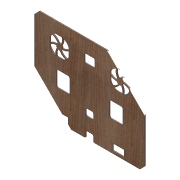
# Autodesk Inventor part: BackCover
Saved by Autodesk Inventor 2015 (Build 190159000, 159)
## iProperties
Created: 2018-04-12
Part Number: BackCover
Material: Wood (Birch)
Document SubType Name: Modeling
Designer: Ghassan Yusuf
Density: 0.55 g/cm^3
Appearance: Birch - Natural Polished
Author: Ghassan Yusuf
Autodesk Inventor part; units mm, degrees
ref_plane "YZ Plane" through (0, 0, 0) normal (1, 0, 0) x (0, 1, 0)
ref_plane "XZ Plane" through (0, 0, 0) normal (0, 1, 0) x (-1, 0, 0)
ref_plane "XY Plane" through (0, 0, 0) normal (0, 0, 1) x (1, 0, 0)
sketch "80 mm Cooling Fan Cut Template" plane through (0, 0, 0) normal (0, 0, 1) x (1, 0, 0)
  line L0 (-145.6797, 134) -> (-114.1203, 134)
  line L1 (-89.9, 109.7797) -> (-89.9, 78.2203)
  line L2 (-114.1203, 54) -> (-145.6797, 54)
  line L3 (-169.9, 78.2203) -> (-169.9, 109.7797)
  circle A0 centre (-165.65, 129.75) radius 2.35
  circle A1 centre (-94.15, 129.75) radius 2.35
  circle A2 centre (-165.65, 58.25) radius 2.35
  circle A3 centre (-94.15, 58.25) radius 2.35
  arc A4 (-89.9, 109.7797) -> (-114.1203, 134) centre (-129.9, 94) ccw
  arc A5 (-145.6797, 134) -> (-169.9, 109.7797) centre (-129.9, 94) ccw
  arc A6 (-169.9, 78.2203) -> (-145.6797, 54) centre (-129.9, 94) ccw
  arc A7 (-114.1203, 54) -> (-89.9, 78.2203) centre (-129.9, 94) ccw
  point P0 (-127.7378, 96.1622)
  point P1 (-129.9, 134)
  point P2 (-89.9, 94)
  dimension "d46" = 4.7
  dimension "d47" = 71.5
  dimension "d48" = 71.5
  dimension "d49" = 4.25
  dimension "d50" = 4.25
  dimension "d52" = 80
  dimension "d53" = 80
  measures "d46" diameter of A0
  measures "d47" distance of A1.centre A0.centre
  measures "d48" distance of A2.centre A0.centre
  measures "d49" distance from line of L0 A0.centre
  measures "d50" distance from line of L3 A0.centre
  measures "d52" distance between parallel lines of L1 L3
  measures "d53" distance between parallel lines of L2 L0
sketch "Faces Holing" plane through (0, 0, 0) normal (0, 0, 1) x (1, 0, 0)
  circle A0 centre (-222, 150) radius 3
  circle A1 centre (-222, 5) radius 3
  circle A2 centre (-222, -150) radius 3
  circle A3 centre (222, -150) radius 3
  circle A4 centre (222, 5) radius 3
  circle A5 centre (222, 150) radius 3
  circle A6 centre (0, 160) radius 3
  circle A7 centre (0, -150) radius 3
  point P0 (0, 2.5)
  dimension "d60" = 6
  dimension "d61" = 145
  dimension "d62" = 155
  measures "d60" diameter of A0
  measures "d61" distance of A4.centre A5.centre
  measures "d62" distance of A3.centre A4.centre
sketch "80 mm Cooling Fan Cut Template_1" plane through (0, 0, 0) normal (0, 0, 1) x (1, 0, 0)
  arc A0 (-145.6797, 134) -> (-169.9, 109.7797) centre (-129.9, 94) ccw
  arc A1 (-114.1203, 54) -> (-89.9, 78.2203) centre (-129.9, 94) ccw
  circle A2 centre (-165.65, 129.75) radius 2.35
  circle A3 centre (-94.15, 129.75) radius 2.35
  circle A4 centre (-165.65, 58.25) radius 2.35
  circle A5 centre (-94.15, 58.25) radius 2.35
  arc A6 (-98.8905, 123.7895) -> (-123.8985, 104.965) centre (-90.5696, 86.7117) ccw
  arc A7 (-102.3594, 127.023) -> (-127.7177, 106.308) centre (-90.5696, 86.7117) ccw
  arc A8 (-140.1937, 135.7497) -> (-136.3952, 104.68) centre (-103.9229, 124.417) ccw
  arc A9 (-144.7285, 134.3623) -> (-139.4679, 102.0439) centre (-103.9229, 124.417) ccw
  arc A10 (-171.2032, 105.9602) -> (-142.3967, 93.7149) centre (-143.2534, 131.7053) ccw
  arc A11 (-172.269, 101.3393) -> (-141.6502, 89.7359) centre (-143.2534, 131.7053) ccw
  arc A12 (-160.9095, 64.2105) -> (-135.9015, 83.035) centre (-169.2304, 101.2883) ccw
  arc A13 (-157.4406, 60.977) -> (-132.0823, 81.692) centre (-169.2304, 101.2883) ccw
  arc A14 (-119.6063, 52.2503) -> (-123.4048, 83.32) centre (-155.8771, 63.583) ccw
  arc A15 (-115.0715, 53.6377) -> (-120.3321, 85.9561) centre (-155.8771, 63.583) ccw
  arc A16 (-88.5968, 82.0398) -> (-117.4033, 94.2851) centre (-116.5466, 56.2947) ccw
  arc A17 (-87.531, 86.6607) -> (-118.1498, 98.2641) centre (-116.5466, 56.2947) ccw
  arc A18 (-89.9, 109.7797) -> (-98.8905, 123.7895) centre (-129.9, 94) ccw
  arc A19 (-102.3594, 127.023) -> (-114.1203, 134) centre (-129.9, 94) ccw
  line L0 (-145.6797, 134) -> (-144.8151, 134)
  line L1 (-140.6948, 134) -> (-114.1203, 134)
  line L2 (-169.9, 78.2203) -> (-169.9, 99.2406)
  line L3 (-169.9, 104.6137) -> (-169.9, 109.7797)
  arc A20 (-169.9, 78.2203) -> (-160.9095, 64.2105) centre (-129.9, 94) ccw
  arc A21 (-157.4406, 60.977) -> (-145.6797, 54) centre (-129.9, 94) ccw
  line L4 (-114.1203, 54) -> (-114.9849, 54)
  line L5 (-119.1052, 54) -> (-145.6797, 54)
  line L6 (-89.9, 109.7797) -> (-89.9, 88.7594)
  line L7 (-89.9, 83.3863) -> (-89.9, 78.2203)
  arc A22 (-118.1498, 98.2641) -> (-123.8985, 104.965) centre (-129.9, 94) ccw
  arc A23 (-127.7177, 106.308) -> (-136.3952, 104.68) centre (-129.9, 94) ccw
  arc A24 (-139.4679, 102.0439) -> (-142.3967, 93.7149) centre (-129.9, 94) ccw
  arc A25 (-141.6502, 89.7359) -> (-135.9015, 83.035) centre (-129.9, 94) ccw
  arc A26 (-132.0823, 81.692) -> (-123.4048, 83.32) centre (-129.9, 94) ccw
  arc A27 (-120.3321, 85.9561) -> (-117.4033, 94.2851) centre (-129.9, 94) ccw
  point P0 (-127.7378, 96.1622)
  point P1 (-129.9, 134)
  point P2 (-89.9, 94)
  dimension "d88" = 4.7
  dimension "d89" = 71.5
  dimension "d90" = 71.5
  dimension "d104" = 4
  dimension "d107" = 360
  measures "d88" diameter of A2
  measures "d89" distance of A3.centre A2.centre
  measures "d90" distance of A4.centre A2.centre
  measures "d104" radial gap between concentric circles of A6 A7
sketch "Sketch1" plane through (0, 0, 0) normal (0, 0, 1) x (1, 0, 0)
  line L0 (-230, 180) -> (230, 180)
  line L1 (230, 180) -> (230, -180)
  line L2 (230, -180) -> (-230, -180)
  line L3 (-230, -180) -> (-230, 180)
  line L4 (-21.9, 125) -> (21.9, 125)
  line L5 (21.9, 125) -> (21.9, 89)
  line L6 (21.9, 89) -> (-21.9, 89)
  line L7 (-21.9, 89) -> (-21.9, 125)
  line L8 (-139.5, 8) -> (-82.5, 8)
  line L9 (-82.5, 8) -> (-82.5, -58.6)
  line L10 (-82.5, -58.6) -> (-139.5, -58.6)
  line L11 (-139.5, -58.6) -> (-139.5, 8)
  line L12 (82.5, 8) -> (139.5, 8)
  line L13 (139.5, 8) -> (139.5, -58.6)
  line L14 (139.5, -58.6) -> (82.5, -58.6)
  line L15 (82.5, -58.6) -> (82.5, 8)
  line L16 (-16.075, -71) -> (16.075, -71)
  line L17 (16.075, -71) -> (16.075, -100.45)
  line L18 (16.075, -100.45) -> (-16.075, -100.45)
  line L19 (-16.075, -100.45) -> (-16.075, -71)
  point P0 (0, 0)
  point P1 (0, 180)
  point P2 (-230, 0)
  point P3 (0, 125)
  point P4 (0, -71)
  point P5 (0, -147)
  dimension "d0" = 460
  dimension "d1" = 360
  dimension "d2" = 55
  dimension "d3" = 43.8
  dimension "d4" = 36
  dimension "d5" = 29.45
  dimension "d6" = 32.15
  dimension "d7" = 66.6
  dimension "d8" = 57
  dimension "d9" = 172
  dimension "d10" = 165
  dimension "d11" = 160
  dimension "d41" = 82.5
  constraints: 40 end point, 10 parallel, 5 horizontal, 5 perpendicular, 4 midpoint, 4 vertical alignment, 2 equal length, 1 horizontal alignment, 1 point on line
  measures "d0" distance of L1.end L2.end
  measures "d1" distance of L0.end L1.end
  measures "d2" distance between parallel lines of L0 L4
  measures "d3" distance of L5.end L6.end
  measures "d4" distance of L6.end L4.start
  measures "d5" distance between parallel lines of L18 L16
  measures "d6" distance of L17.end L18.end
  measures "d7" distance between parallel lines of L10 L8
  measures "d8" distance between parallel lines of L9 L11
  measures "d9" distance between parallel lines of L8 L0
  measures "d10" distance between parallel lines of L15 L9
  measures "d11" distance between parallel lines of L16 L6
  measures "d41" distance from line of point (0, 0) L15
extrude "Shape Cut" add sketch "Sketch1" against normal blind 4
chamfer "Outer Frame Chamfer" distance 20 angle 45 4 edges at (-230, 180, -2) (230, 180, -2) (230, -180, -2) (-230, -180, -2)
fillet "Outer Frame Coner Fillet" radius 5 8 edges at (-230, 160, -2) (-210, 180, -2) (210, 180, -2) (230, 160, -2) (230, -160, -2) (210, -180, -2) (-210, -180, -2) (-230, -160, -2)
fillet "Cable Guide Cut Fillet" radius 5 8 edges at (-21.9, 125, -2) (-21.9, 89, -2) (21.9, 125, -2) (21.9, 89, -2) (-16.075, -71, -2) (-16.075, -100.45, -2) (16.075, -71, -2) (16.075, -100.45, -2)
sketch "Sketch3" plane through (0, 0, -4) normal (0, 0, -1) x (-1, 0, 0)
  line L0 (-144, -142.8) -> (-96.65, -142.8)
  line L1 (-96.65, -142.8) -> (-96.65, -170)
  line L2 (-96.65, -170) -> (-144, -170)
  line L3 (-144, -170) -> (-144, -142.8)
  line L4 (-207.9289, -180) -> (207.9289, -180) projected
  line L5 (-230, 157.9289) -> (-230, -157.9289) projected
  point P0 (0, 0)
  dimension "d29" = 10
  dimension "d30" = 27.2
  dimension "d31" = 47.35
  dimension "d32" = 86
  constraints: 8 end point, 2 parallel, 1 horizontal, 1 perpendicular
  measures "d29" distance between parallel lines of L4 L2
  measures "d30" distance between parallel lines of L2 L0
  measures "d31" distance between parallel lines of L1 L3
  measures "d32" distance between parallel lines of L5 L3
extrude "240V Power Line Connector" cut sketch "Sketch3" against normal blind 5
sketch "Sketch4" plane through (0, 0, -4) normal (0, 0, -1) x (-1, 0, 0)
  line L0 (89, -170) -> (189, -170)
  line L1 (189, -170) -> (189, -142.8)
  line L2 (189, -142.8) -> (89, -142.8)
  line L3 (89, -142.8) -> (89, -170)
  line L4 (230, -157.9289) -> (230, 157.9289) projected
  line L5 (-207.9289, -180) -> (207.9289, -180) projected
  line L6 (-16.075, -180) -> (16.075, -180)
  line L7 (16.075, -180) -> (16.075, -152.8)
  line L8 (16.075, -152.8) -> (-16.075, -152.8)
  line L9 (-16.075, -152.8) -> (-16.075, -180)
  line L10 (11.075, -100.45) -> (-11.075, -100.45) projected
  line L11 (16.075, -76) -> (16.075, -95.45) projected
  line L12 (-144, -142.8) -> (-96.65, -142.8) projected
  point P0 (0, 0)
  point P1 (0, -152.8)
  point P2 (0, -100.45)
  dimension "d35" = 41
  dimension "d36" = 100
  dimension "d37" = 27.2
  constraints: 16 end point, 5 parallel, 2 collinear, 2 horizontal, 2 midpoint, 2 perpendicular, 1 point on line, 1 vertical alignment
  measures "d35" distance between parallel lines of L4 L1
  measures "d36" distance of L1.end L2.end
  measures "d37" distance of L2.end L0.start
extrude "Electronic Board Frame Cut" cut sketch "Sketch4" against normal blind 5
fillet "Fillet3" radius 5 4 edges at (-16.075, -180, -2) (-16.075, -152.8, -2) (16.075, -152.8, -2) (16.075, -180, -2)
sketch "Sketch5" plane through (0, 0, 0) normal (0, 0, 1) x (1, 0, 0)
  line L0 (-21.9, 94) -> (-21.9, 120) projected
  line L1 (21.9, 120) -> (21.9, 94) projected
  line L2 (0, 0) -> (0, 178.9136)
  arc A0 (110.1203, 134) -> (85.9, 109.7797) centre (125.9, 94) ccw
  arc A1 (141.6797, 54) -> (165.9, 78.2203) centre (125.9, 94) ccw
  circle A2 centre (90.15, 129.75) radius 2.35
  circle A3 centre (161.65, 129.75) radius 2.35
  circle A4 centre (90.15, 58.25) radius 2.35
  circle A5 centre (161.65, 58.25) radius 2.35
  arc A6 (156.9095, 123.7895) -> (131.9015, 104.965) centre (165.2304, 86.7117) ccw
  arc A7 (153.4406, 127.023) -> (128.0823, 106.308) centre (165.2304, 86.7117) ccw
  arc A8 (115.6063, 135.7497) -> (119.4048, 104.68) centre (151.8771, 124.417) ccw
  arc A9 (111.0715, 134.3623) -> (116.3321, 102.0439) centre (151.8771, 124.417) ccw
  arc A10 (84.5968, 105.9602) -> (113.4033, 93.7149) centre (112.5466, 131.7053) ccw
  arc A11 (83.531, 101.3393) -> (114.1498, 89.7359) centre (112.5466, 131.7053) ccw
  arc A12 (94.8905, 64.2105) -> (119.8985, 83.035) centre (86.5696, 101.2883) ccw
  arc A13 (98.3594, 60.977) -> (123.7177, 81.692) centre (86.5696, 101.2883) ccw
  arc A14 (136.1937, 52.2503) -> (132.3952, 83.32) centre (99.9229, 63.583) ccw
  arc A15 (140.7285, 53.6377) -> (135.4679, 85.9561) centre (99.9229, 63.583) ccw
  arc A16 (167.2032, 82.0398) -> (138.3967, 94.2851) centre (139.2534, 56.2947) ccw
  arc A17 (168.269, 86.6607) -> (137.6502, 98.2641) centre (139.2534, 56.2947) ccw
  arc A18 (165.9, 109.7797) -> (156.9095, 123.7895) centre (125.9, 94) ccw
  arc A19 (153.4406, 127.023) -> (141.6797, 134) centre (125.9, 94) ccw
  line L3 (110.1203, 134) -> (110.9849, 134)
  line L4 (115.1052, 134) -> (141.6797, 134)
  line L5 (85.9, 78.2203) -> (85.9, 99.2406)
  line L6 (85.9, 104.6137) -> (85.9, 109.7797)
  arc A20 (85.9, 78.2203) -> (94.8905, 64.2105) centre (125.9, 94) ccw
  arc A21 (98.3594, 60.977) -> (110.1203, 54) centre (125.9, 94) ccw
  line L7 (141.6797, 54) -> (140.8151, 54)
  line L8 (136.6948, 54) -> (110.1203, 54)
  line L9 (165.9, 109.7797) -> (165.9, 88.7594)
  line L10 (165.9, 83.3863) -> (165.9, 78.2203)
  arc A22 (137.6502, 98.2641) -> (131.9015, 104.965) centre (125.9, 94) ccw
  arc A23 (128.0823, 106.308) -> (119.4048, 104.68) centre (125.9, 94) ccw
  arc A24 (116.3321, 102.0439) -> (113.4033, 93.7149) centre (125.9, 94) ccw
  arc A25 (114.1498, 89.7359) -> (119.8985, 83.035) centre (125.9, 94) ccw
  arc A26 (123.7177, 81.692) -> (132.3952, 83.32) centre (125.9, 94) ccw
  arc A27 (135.4679, 85.9561) -> (138.3967, 94.2851) centre (125.9, 94) ccw
  arc A28 (-110.1203, 134) -> (-85.9, 109.7797) centre (-125.9, 94) cw
  arc A29 (-141.6797, 54) -> (-165.9, 78.2203) centre (-125.9, 94) cw
  circle A30 centre (-90.15, 129.75) radius 2.35
  circle A31 centre (-161.65, 129.75) radius 2.35
  circle A32 centre (-90.15, 58.25) radius 2.35
  circle A33 centre (-161.65, 58.25) radius 2.35
  arc A34 (-156.9095, 123.7895) -> (-131.9015, 104.965) centre (-165.2304, 86.7117) cw
  arc A35 (-153.4406, 127.023) -> (-128.0823, 106.308) centre (-165.2304, 86.7117) cw
  arc A36 (-115.6063, 135.7497) -> (-119.4048, 104.68) centre (-151.8771, 124.417) cw
  arc A37 (-111.0715, 134.3623) -> (-116.3321, 102.0439) centre (-151.8771, 124.417) cw
  arc A38 (-84.5968, 105.9602) -> (-113.4033, 93.7149) centre (-112.5466, 131.7053) cw
  arc A39 (-83.531, 101.3393) -> (-114.1498, 89.7359) centre (-112.5466, 131.7053) cw
  arc A40 (-94.8905, 64.2105) -> (-119.8985, 83.035) centre (-86.5696, 101.2883) cw
  arc A41 (-98.3594, 60.977) -> (-123.7177, 81.692) centre (-86.5696, 101.2883) cw
  arc A42 (-136.1937, 52.2503) -> (-132.3952, 83.32) centre (-99.9229, 63.583) cw
  arc A43 (-140.7285, 53.6377) -> (-135.4679, 85.9561) centre (-99.9229, 63.583) cw
  arc A44 (-167.2032, 82.0398) -> (-138.3967, 94.2851) centre (-139.2534, 56.2947) cw
  arc A45 (-168.269, 86.6607) -> (-137.6502, 98.2641) centre (-139.2534, 56.2947) cw
  arc A46 (-165.9, 109.7797) -> (-156.9095, 123.7895) centre (-125.9, 94) cw
  arc A47 (-153.4406, 127.023) -> (-141.6797, 134) centre (-125.9, 94) cw
  line L11 (-110.1203, 134) -> (-110.9849, 134)
  line L12 (-115.1052, 134) -> (-141.6797, 134)
  line L13 (-85.9, 78.2203) -> (-85.9, 99.2406)
  line L14 (-85.9, 104.6137) -> (-85.9, 109.7797)
  arc A48 (-85.9, 78.2203) -> (-94.8905, 64.2105) centre (-125.9, 94) cw
  arc A49 (-98.3594, 60.977) -> (-110.1203, 54) centre (-125.9, 94) cw
  line L15 (-141.6797, 54) -> (-140.8151, 54)
  line L16 (-136.6948, 54) -> (-110.1203, 54)
  line L17 (-165.9, 109.7797) -> (-165.9, 88.7594)
  line L18 (-165.9, 83.3863) -> (-165.9, 78.2203)
  arc A50 (-137.6502, 98.2641) -> (-131.9015, 104.965) centre (-125.9, 94) cw
  arc A51 (-128.0823, 106.308) -> (-119.4048, 104.68) centre (-125.9, 94) cw
  arc A52 (-116.3321, 102.0439) -> (-113.4033, 93.7149) centre (-125.9, 94) cw
  arc A53 (-114.1498, 89.7359) -> (-119.8985, 83.035) centre (-125.9, 94) cw
  arc A54 (-123.7177, 81.692) -> (-132.3952, 83.32) centre (-125.9, 94) cw
  arc A55 (-135.4679, 85.9561) -> (-138.3967, 94.2851) centre (-125.9, 94) cw
  dimension "d109" = 64
  dimension "d110" = 94
  constraints: 2 end point, 2 vertical
extrude "Extrusion5" cut sketch "Sketch5" against normal blind 10
sketch "Sketch6" plane through (0, 0, -4) normal (0, 0, -1) x (-1, 0, 0)
  line L0 (-207.9289, -180) -> (207.9289, -180) projected
  circle A0 centre (-121, -136.4) radius 1.6
  circle A1 centre (-121, -176.4) radius 1.6
  line L1 (-144, -142.8) -> (-96.65, -142.8) projected
  line L2 (-144, -170) -> (-144, -142.8) projected
  circle A2 centre (-222, 150) radius 3
  circle A3 centre (-222, 5) radius 3
  circle A4 centre (-222, -150) radius 3
  circle A5 centre (222, -150) radius 3
  circle A6 centre (222, 5) radius 3
  circle A7 centre (222, 150) radius 3
  circle A8 centre (0, 160) radius 3
  circle A9 centre (0, -150) radius 3
  point P0 (0, 0)
  point P1 (84, -180)
  dimension "d63" = 30
  dimension "d67" = 3.2
  dimension "d68" = 40
  dimension "d70" = 23
  dimension "d71" = 6.4
  constraints: 2 centre point, 1 equal radius, 1 vertical alignment, 1 other
  measures "d67" diameter of A0
  measures "d68" distance of A1.centre A0.centre
  measures "d70" distance from line of A0.centre L2
  measures "d71" distance from line of L1 A0.centre
extrude "Extrusion6" cut sketch "Sketch6" against normal blind 10 contours A0 | A1 | A2 | A3 | A4 | A5 | A6 | A7 | A8
chamfer "Chamfer3" distance 5 angle 45 8 edges at (139.5, 8, -2) (82.5, 8, -2) (139.5, -58.6, -2) (82.5, -58.6, -2) (-82.5, 8, -2) (-82.5, -58.6, -2) (-139.5, -58.6, -2) (-139.5, 8, -2)
equation "\"d41\" = 0.5 * d10"
equation "\"d49\" = -0.5 * d48 + 0.5 * d42"
equation "\"d50\" = d49"
equation "\"d91\" = -0.5 * d90 + 0.5 * d95"
equation "\"d92\" = d91"
equation "\"d42\" = 80"
equation "\"d95\" = 80"
body "Solid1"
